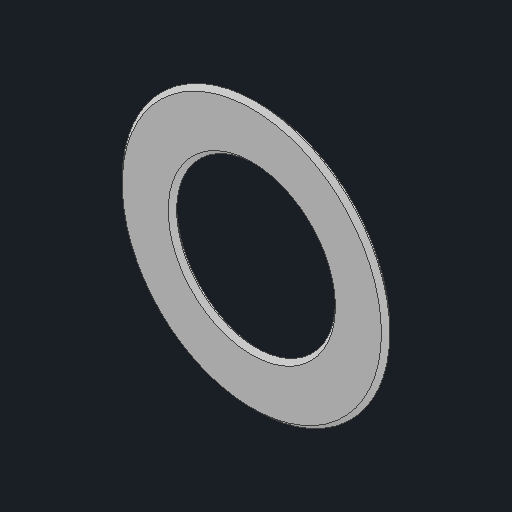
# Autodesk Inventor part: Bottom_Ring
Saved by Autodesk Inventor 2024 (Build 280153000, 153)
## iProperties
Created: 2023-08-24
Part Number: Bottom_Ring
Material: Generic
Document SubType Name: Modeling
Designer: Izack Waczko
Density: 1 g/cm^3
Appearance: Default
Author: Izack Waczko
Autodesk Inventor part; units mm, degrees
ref_plane "YZ Plane" through (0, 0, 0) normal (1, 0, 0) x (0, 1, 0)
ref_plane "XZ Plane" through (0, 0, 0) normal (0, 1, 0) x (-1, 0, 0)
ref_plane "XY Plane" through (0, 0, 0) normal (0, 0, 1) x (1, 0, 0)
sketch "Sketch1" plane through (0, 0, 0) normal (0, 0, 1) x (1, 0, 0)
  circle A0 centre (0, 0) radius 23.75
  circle A1 centre (0, 0) radius 40
  dimension "d0" = 47.5
  dimension "d1" = 80
  constraints: 2 centre point, 2 coincident
  measures "d0" diameter of A0
  measures "d1" diameter of A1
extrude "Extrusion1" add sketch "Sketch1" along normal blind 2.5
chamfer "Chamfer1" distance 1.25 angle 45 4 edges at (-40, 0, 0) (-40, 0, 2.5) (-23.75, 0, 2.5) (-23.75, 0, 0)
body "Solid1"
